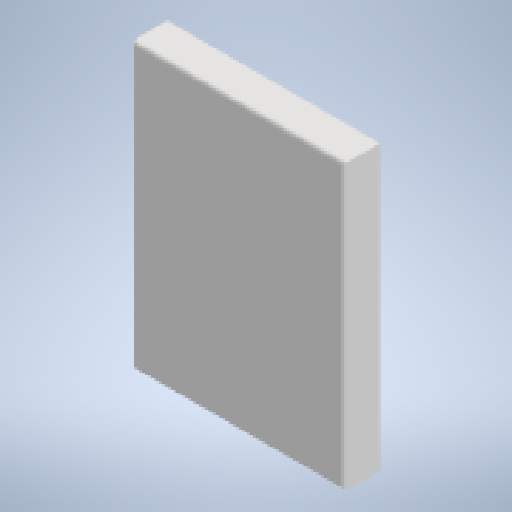
# Autodesk Inventor part: Mattress
Saved by Autodesk Inventor 2024 (Build 280153000, 153)
## iProperties
Created: 2024-10-17
Part Number: Mattress
Material: 一般
Document SubType Name: Modeling
Designer: jerry
Density: 1 g/cm^3
Appearance: 預設
Author: jerry
Autodesk Inventor part; units mm, degrees
ref_plane "YZ Plane" through (0, 0, 0) normal (1, 0, 0) x (0, 1, 0)
ref_plane "XZ Plane" through (0, 0, 0) normal (0, 1, 0) x (-1, 0, 0)
ref_plane "XY Plane" through (0, 0, 0) normal (0, 0, 1) x (1, 0, 0)
sketch "草圖1" plane through (0, 0, 0) normal (0, 0, 1) x (1, 0, 0)
  circle A0 centre (0, 0) radius 50
  line L0 (250, 400) -> (-350, 400)
  line L1 (-350, 400) -> (-350, -400)
  line L2 (-350, -400) -> (250, -400)
  line L3 (250, -400) -> (250, 400)
  line L4 (250, 400) -> (-350, -400) construction
  line L5 (-350, 400) -> (250, -400) construction
  point P0 (-50, 0)
  dimension "d0" = 100
  dimension "d1" = 600
  dimension "d2" = 800
  constraints: 12 end point, 2 midpoint, 2 parallel, 1 coincident, 1 horizontal, 1 horizontal alignment, 1 perpendicular, 2 other
  measures "d1" distance of L2.end L1.end
  measures "d2" distance of L1.end L0.end
extrude "擠出1" add sketch "草圖1" along normal blind 100 contours A0 | L3 L2 L1 L0
fillet "圓角1" radius 10 4 edges at (250, 0, 100) (-50, 400, 100) (-50, -400, 100) (-350, 0, 100)
